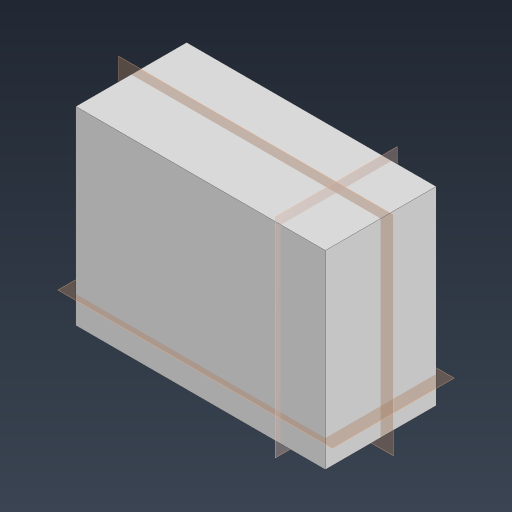
# Autodesk Inventor part: Козырёк_версия_2
Saved by Autodesk Inventor 2023.2 (Build 272271030, 271C)
## iProperties
Created: 2025-10-07
Part Number: Козырёк_версия_2
Material: Типовые
Document SubType Name: Modeling
Designer: Олег Коноваленко
Density: 1 g/cm^3
Appearance: По умолчанию
Author: Олег Коноваленко
Autodesk Inventor part; units mm, degrees
sketch "Эскиз1" plane through (0, 0, 0) normal (0, 0, 1) x (1, 0, 0)
  line L0 (-18.4957, 14.6641) -> (4.0208, 14.6641)
  line L1 (4.0208, 14.6641) -> (4.0208, -2.4598)
  line L2 (4.0208, -2.4598) -> (-18.4957, -2.4598)
  line L3 (-18.4957, -2.4598) -> (-18.4957, 14.6641)
  line L4 (-18.4957, 14.6641) -> (4.0208, -2.4598) construction
  line L5 (4.0208, 14.6641) -> (-18.4957, -2.4598) construction
  point P0 (0, 0)
  point P1 (-7.2375, 6.1022)
  constraints: 12 end point, 2 midpoint, 2 parallel, 1 horizontal, 1 perpendicular
extrude "Выдавливание1" add sketch "Эскиз1" along normal mid plane 10
